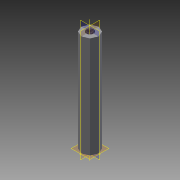
# Autodesk Inventor part: LenkungStütze
Saved by Autodesk Inventor 2015 (Build 190159000, 159)
## iProperties
Created: 2018-10-20
Part Number: LenkungStütze
Material: Generisch
Document SubType Name: Modeling
Designer: Boris
Density: 1 g/cm^3
Appearance: Vorgabe
Author: Boris
Autodesk Inventor part; units mm, degrees
sketch "Skizze1" plane through (0, 0, 0) normal (0, 0, 1) x (1, 0, 0)
  line L0 (0, 4.9) -> (0, -4.9) projected
  line L1 (-4.9, 0) -> (4.9, 0) projected
  line L2 (0, 3.5) -> (2.4749, 2.4749)
  line L3 (2.4749, 2.4749) -> (3.5, 0)
  line L4 (3.5, 0) -> (2.4749, -2.4749)
  line L5 (2.4749, -2.4749) -> (0, -3.5)
  line L6 (0, -3.5) -> (-2.4749, -2.4749)
  line L7 (-2.4749, -2.4749) -> (-3.5, 0)
  line L8 (-3.5, 0) -> (-2.4749, 2.4749)
  line L9 (-2.4749, 2.4749) -> (0, 3.5)
  circle A0 centre (0, 0) radius 1.5
  dimension "d1" = 3
  constraints: 16 end point, 1 centre point, 1 coincident, 1 point on line, 17 other
  measures "d1" diameter of A0
extrude "Extrusion1" add sketch "Skizze1" along normal blind 41.5 contours L2 L3 L1 A0 L0 | L0 A0 L1 L8 L9 | L1 L4 L5 L0 A0 | A0 L0 L6 L7 L1
thread "Gewinde1" size "M3x0.5" class "6H" standard "ANSI Metric M Profile" full length
